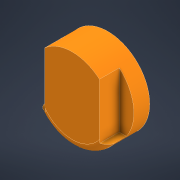
# Autodesk Inventor part: 02_DoF1_Podstawa
Saved by Autodesk Inventor 2022 (Build 260153000, 153)
## iProperties
Created: 2022-05-07
Part Number: 02_DoF1_Podstawa
Material: Generic
Document SubType Name: Modeling
Designer: pzach
Density: 1 g/cm^3
Appearance: Orange
Author: pzach
Autodesk Inventor part; units mm, degrees
ref_plane "YZ Plane" through (0, 0, 0) normal (1, 0, 0) x (0, 1, 0)
ref_plane "XZ Plane" through (0, 0, 0) normal (0, 1, 0) x (-1, 0, 0)
ref_plane "XY Plane" through (0, 0, 0) normal (0, 0, 1) x (1, 0, 0)
sketch "Sketch1" plane through (0, 0, 0) normal (0, 0, 1) x (1, 0, 0)
  circle A0 centre (0, 0) radius 530
  dimension "d0" = 1060
  constraints: 1 centre point, 1 coincident
  measures "d0" diameter of A0
extrude "Extrusion1" add sketch "Sketch1" along normal blind 200
sketch "Sketch2" plane through (0, 0, 200) normal (0, 0, 1) x (1, 0, 0)
  circle A0 centre (0, 0) radius 530 projected
  line L0 (0, 0) -> (0, -300) construction
  line L1 (436.921, -300) -> (-436.921, -300)
  line L2 (-344.9012, -300) -> (-344.9012, 402.4216)
  line L3 (344.9012, -300) -> (344.9012, 402.4216)
  dimension "d3" = 300
  dimension "d5" = 873.8421
  dimension "d14" = 344.9012
  constraints: 8 end point, 3 point on circle, 2 symmetric about line, 2 vertical, 1 horizontal, 1 point on line
  measures "d3" distance of L0.start L0.end
  measures "d5" distance of L1.start L1.end
  measures "d14" distance from line of L0.end L2
extrude "Extrusion2" add sketch "Sketch2" along normal blind 250 contours L3 L1 L2 A0 | A0 L1
fillet "Fillet1" radius 100 1 edges at (0, -530, 450)
equation "\"d6\" = d9"
equation "\"d9\" = 250"
body "Solid1"
